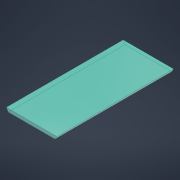
# Autodesk Inventor part: watah
Saved by Autodesk Inventor 2022 (Build 260153000, 153)
## iProperties
Created: 2022-02-21
Part Number: watah
Material: Generic
Document SubType Name: Modeling
Designer: Lukas
Density: 1 g/cm^3
Appearance: Indoor Pool
Author: Lukas
Autodesk Inventor part; units mm, degrees
ref_plane "YZ Plane" through (0, 0, 0) normal (1, 0, 0) x (0, 1, 0)
ref_plane "XZ Plane" through (0, 0, 0) normal (0, 1, 0) x (-1, 0, 0)
ref_plane "XY Plane" through (0, 0, 0) normal (0, 0, 1) x (1, 0, 0)
sketch "Sketch1" plane through (0, 0, 0) normal (0, 0, 1) x (1, 0, 0)
  line L0 (0, 0) -> (2000, 0)
  line L1 (0, 0) -> (-79.9516, 138.592)
  line L2 (0, 0) -> (160, 0) construction
  line L3 (2000, 0) -> (2079.5158, 138.8425)
  line L4 (2000, 0) -> (2160, 0) construction
  line L5 (-79.9516, 138.592) -> (2079.5158, 138.8425)
  dimension "d0" = 2000
  dimension "d1" = 160
  dimension "d2" = 119.98
  dimension "d3" = 160
  dimension "d4" = 60.2
  dimension "d5" = 2159.4675
  constraints: 12 end point, 3 horizontal, 2 equal length
  measures "d0" distance of L0.start L0.end
  measures "d1" distance of L0.start L1.end
  measures "d2" angle of L2 L1
  measures "d3" distance of L0.end L3.end
  measures "d4" angle of L4 L3
  measures "d5" distance of L1.end L3.end
extrude "Extrusion1" add sketch "Sketch1" against normal blind 5000
body "Solid1"
